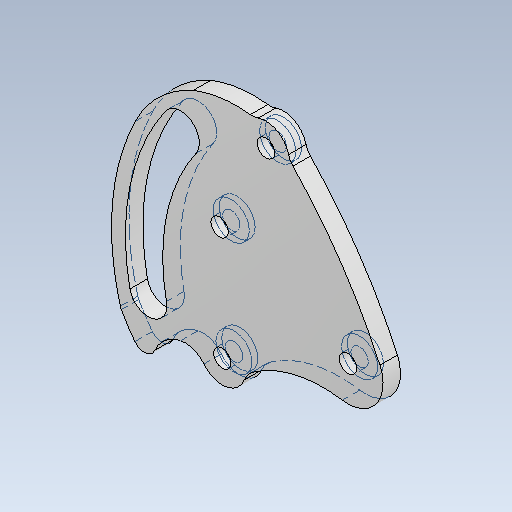
# Autodesk Inventor part: アンノーン前
Saved by Autodesk Inventor 2020 (Build 240168000, 168)
## iProperties
Created: 2021-02-23
Part Number: アンノーン前
Material: アルミニウム 2014-T4
Document SubType Name: Modeling
Designer: AA19065
Density: 2.8 g/cm^3
Appearance: サテン
Mass: 9.74033 g
Surface Area: 32.1311 cm^2
Volume: 3.47869 cm^3
Author: AA19065
Autodesk Inventor part; units mm, degrees
ref_plane "YZ Plane" through (0, 0, 0) normal (1, 0, 0) x (0, 1, 0)
ref_plane "XZ Plane" through (0, 0, 0) normal (0, 1, 0) x (-1, 0, 0)
ref_plane "XY Plane" through (0, 0, 0) normal (0, 0, 1) x (1, 0, 0)
sketch "スケッチ1" plane through (0, 0, 0) normal (0, 0, 1) x (1, 0, 0)
  line L0 (108, 72.831817) -> (108, -27.637331) construction
  circle A0 centre (90, 27) radius 3
  circle A1 centre (104.07345, 2) radius 6.025
  circle A2 centre (90, 27) radius 1.5
  circle A3 centre (104.07345, 2) radius 1.5
  circle A4 centre (82.04031, 11.281864) radius 1.5
  circle A5 centre (82.5, -8) radius 3
  circle A6 centre (82.5, -8) radius 1.5
  arc A7 (66.645247, -5.64) -> (72.915941, -4.36) centre (69.780594, -5) ccw
  arc A8 (72.724551, 23.828571) -> (66.645247, -5.64) centre (104.07345, 2) ccw
  arc A9 (77.976723, 20.171429) -> (72.915941, -4.36) centre (104.07345, 2) ccw
  arc A10 (77.976723, 20.171429) -> (72.724551, 23.828571) centre (75.350637, 22) ccw
  circle A11 centre (137.322151, 20) radius 1.25
  circle A12 centre (133.5, -8) radius 3
  circle A13 centre (133.5, -8) radius 1.5
  circle A14 centre (146, 10) radius 1.5
  arc A15 (-6.089587, 13.373015) -> (73.990447, 1.93301) centre (42.288654, 66.020578) ccw construction
  line L1 (108, 72.831817) -> (108, -27.637331) construction
  arc A16 (142.009553, 1.93301) -> (222.089587, 13.373015) centre (173.711346, 66.020578) ccw construction
  arc A17 (142.29705, -19.072921) -> (142.660887, 27.253552) centre (125.709293, 4.222021) ccw
  arc A18 (136.80781, 35.127338) -> (180.06622, 10.718677) centre (180.861669, 62.665248) ccw
  circle A19 centre (137.322151, 20) radius 9.006449
  arc A20 (128.322651, 20.353731) -> (130.555913, -8.5765) centre (253.226204, 15.444317) ccw
  arc A21 (133.414591, -10.998784) -> (152.948723, -4.485529) centre (134.268683, 18.989056) ccw
  arc A22 (35.93378, 10.718677) -> (79.19219, 35.127338) centre (35.138331, 62.665248) ccw
  arc A23 (73.339113, 27.253552) -> (73.70295, -19.072921) centre (90.290707, 4.222021) ccw
  arc A24 (90.887703, 29.865656) -> (71.118535, 25.188537) centre (84.969685, 10.761283) ccw
  arc A25 (109.559222, 4.491371) -> (92.075879, 29.165808) centre (36.719095, -28.589074) ccw
  arc A26 (80.567193, -10.294397) -> (70.653319, -16.566942) centre (76.603177, -15) ccw
  circle A27 centre (76.603177, -15) radius 5 construction
  circle A28 centre (94, -11) radius 1.5
  circle A29 centre (94, -11) radius 3
  arc A30 (103.111347, -3.947687) -> (84.657245, -10.084777) centre (99.757959, -24.678215) ccw
  point P0 (0, 0)
  point P1 (0, 0)
  point P2 (153.490711, -2.560367)
  point P3 (70.420594, -8.135347)
  point P4 (68.814065, 23.104865)
  dimension "d0" = 2
  dimension "d1" = 30
  dimension "d2" = 125
  dimension "d3" = 80
  dimension "d4" = 20
  dimension "d5" = 6
  dimension "d6" = 21
  constraints: 47 point on circle, 30 centre point, 10 tangent, 4 end point, 3 symmetric about line, 1 coincident, 1 vertical, 32 other
  measures "d0" distance of point (153.491, -2.56) A21.end
  measures "d1" radius of A21
  measures "d2" radius of A20
  measures "d3" radius of A25
  measures "d4" radius of A24
  measures "d5" diameter of A29
  measures "d6" radius of A30
extrude "押し出し1" add sketch "スケッチ1" along normal blind 3 contours A0 | A0 A25 A1 A30 A5 A26 A23 A22 A24 | A1 | A5
fillet "フィレット1" radius 5 1 edges at (68.8141, 23.1049, 1.5)
fillet "フィレット2" radius 2 1 edges at (70.6533, -16.5669, 1.5)
sketch "スケッチ2" plane through (0, 0, 0) normal (0, 0, -1) x (-1, 0, 0)
  circle A0 centre (-82.04031, 11.281864) radius 1.5
  arc A1 (-70.932275, -12.613165) -> (-67.494617, -13.044892) centre (-69.088898, -11.837303) ccw
  arc A2 (-67.494617, -13.044892) -> (-68.54743, 22.797215) centre (-90.290707, 4.222021) ccw
  arc A3 (-68.54743, 22.797215) -> (-69.082243, 23.334729) centre (-72.349055, 19.549502) ccw
  arc A4 (-71.118535, 25.188537) -> (-69.082243, 23.334729) centre (-35.138331, 62.665248) ccw
  arc A5 (-71.118535, 25.188537) -> (-90.887703, 29.865656) centre (-84.969685, 10.761283) ccw
  arc A6 (-90.887703, 29.865656) -> (-92.075879, 29.165808) centre (-90, 27) ccw
  arc A7 (-92.075879, 29.165808) -> (-109.559222, 4.491371) centre (-36.719095, -28.589074) ccw
  arc A8 (-109.559222, 4.491371) -> (-103.111347, -3.947687) centre (-104.07345, 2) ccw
  arc A9 (-84.657245, -10.084777) -> (-103.111347, -3.947687) centre (-99.757959, -24.678215) ccw
  arc A10 (-84.657245, -10.084777) -> (-80.567193, -10.294397) centre (-82.5, -8) ccw
  arc A11 (-70.932275, -12.613165) -> (-80.567193, -10.294397) centre (-76.603177, -15) ccw
  circle A12 centre (-82.5, -8) radius 1.5
  circle A13 centre (-104.07345, 2) radius 1.5
  circle A14 centre (-90, 27) radius 1.5
  circle A15 centre (-82.04031, 11.281864) radius 1.5
  arc A16 (-72.724551, 23.828571) -> (-77.976723, 20.171429) centre (-75.350637, 22) ccw
  arc A17 (-66.645247, -5.64) -> (-72.724551, 23.828571) centre (-104.07345, 2) ccw
  arc A18 (-72.915941, -4.36) -> (-66.645247, -5.64) centre (-69.780594, -5) ccw
  arc A19 (-72.915941, -4.36) -> (-77.976723, 20.171429) centre (-104.07345, 2) ccw
  circle A20 centre (-90, 27) radius 3.1
  circle A21 centre (-82.04031, 11.281864) radius 3.1
  circle A22 centre (-104.07345, 2) radius 3.1
  circle A23 centre (-82.5, -8) radius 3.1
  arc A24 (-86.256515, -9.37426) -> (-87.720107, -7.470946) centre (-90.013031, -10.748521) ccw
  arc A25 (-86.256515, -9.37426) -> (-79.334786, -10.445694) centre (-82.5, -8) ccw
  arc A26 (-75.363887, -8.973369) -> (-79.334786, -10.445694) centre (-76.169572, -12.891388) ccw
  arc A27 (-70.932275, -12.613165) -> (-80.567193, -10.294397) centre (-76.603177, -15) ccw
  arc A28 (-94.623726, 26.61105) -> (-93.882942, 27.960603) centre (-96.795149, 28.681055) ccw
  arc A29 (-88.670242, 30.772498) -> (-93.882942, 27.960603) centre (-90, 27) ccw
  arc A30 (-88.670242, 30.772498) -> (-87.320327, 30.622665) centre (-87.672923, 33.601872) ccw
  point P0 (0, 0)
  dimension "d11" = 6.2
  dimension "d12" = 6.2
  dimension "d13" = 6.2
  dimension "d14" = 6.2
  dimension "d15" = 4
  dimension "d16" = 4
  dimension "d17" = 4
  dimension "d18" = 4
  dimension "d19" = 3
  dimension "d20" = 3
  constraints: 16 point on circle, 10 centre point, 8 tangent, 4 coincident, 2 concentric
  measures "d11" diameter of A20
  measures "d12" diameter of A21
  measures "d13" diameter of A22
  measures "d14" diameter of A23
  measures "d15" radius of A25
  measures "d16" radius of A26
  measures "d17" radius of A24
  measures "d18" radius of A29
  measures "d19" radius of A30
  measures "d20" radius of A28
extrude "押し出し2" add sketch "スケッチ2" against normal up to surface (3 mm away) contours A26 A25 A24 A9 A23 A11 | A23 A9 A10 A11 | A5 A20 A7 A28 A29 A30 | A5 A6 A7 A20 picked at (-81.994217, -10.979131) picked at (-91.467973, 29.678904)
extrude "押し出し3" cut sketch "スケッチ2" against normal blind 1 contours A23 A9 A10 A11 | A11 A10 A9 A23 | A20 A7 A6 A5 | A5 A6 A7 A20 | A12 | A14 | A21 | A22
sketch "スケッチ4" plane through (0, 0, 3) normal (0, 0, 1) x (1, 0, 0)
  arc A0 (67.494617, -13.044892) -> (70.932275, -12.613165) centre (69.088898, -11.837303) ccw
  arc A1 (75.363887, -8.973369) -> (70.932275, -12.613165) centre (76.603177, -15) ccw
  arc A2 (79.334786, -10.445694) -> (75.363887, -8.973369) centre (76.169572, -12.891388) ccw
  arc A3 (79.334786, -10.445694) -> (86.256515, -9.37426) centre (82.5, -8) ccw
  arc A4 (87.720107, -7.470946) -> (86.256515, -9.37426) centre (90.013031, -10.748521) ccw
  arc A5 (103.111347, -3.947687) -> (87.720107, -7.470946) centre (99.757959, -24.678215) ccw
  arc A6 (103.111347, -3.947687) -> (109.559222, 4.491371) centre (104.07345, 2) ccw
  arc A7 (109.559222, 4.491371) -> (94.623726, 26.61105) centre (36.719095, -28.589074) ccw
  arc A8 (93.882942, 27.960603) -> (94.623726, 26.61105) centre (96.795149, 28.681055) ccw
  arc A9 (93.882942, 27.960603) -> (88.670242, 30.772498) centre (90, 27) ccw
  arc A10 (87.320327, 30.622665) -> (88.670242, 30.772498) centre (87.672923, 33.601872) ccw
  arc A11 (87.320327, 30.622665) -> (71.118535, 25.188537) centre (84.969685, 10.761283) ccw
  arc A12 (69.082243, 23.334729) -> (71.118535, 25.188537) centre (35.138331, 62.665248) ccw
  arc A13 (69.082243, 23.334729) -> (68.54743, 22.797215) centre (72.349055, 19.549502) ccw
  arc A14 (68.54743, 22.797215) -> (67.494617, -13.044892) centre (90.290707, 4.222021) ccw
  circle A15 centre (82.5, -8) radius 1.5
  circle A16 centre (104.07345, 2) radius 1.5
  circle A17 centre (90, 27) radius 1.5
  circle A18 centre (82.04031, 11.281864) radius 1.5
  arc A19 (77.976723, 20.171429) -> (72.724551, 23.828571) centre (75.350637, 22) ccw
  arc A20 (77.976723, 20.171429) -> (72.915941, -4.36) centre (104.07345, 2) ccw
  arc A21 (66.645247, -5.64) -> (72.915941, -4.36) centre (69.780594, -5) ccw
  arc A22 (72.724551, 23.828571) -> (66.645247, -5.64) centre (104.07345, 2) ccw
  arc A23 (70.112674, 24.248139) -> (65.061877, -9.243272) centre (104.07345, 2) ccw
  arc A24 (72.724551, 23.828571) -> (66.645247, -5.64) centre (104.07345, 2) ccw
  arc A25 (77.522944, 29.323235) -> (67.556607, 19.743566) centre (85.545451, 11.002771) ccw
  point P0 (0, 0)
  dimension "d28" = 20
  constraints: 8 point on circle, 2 centre point, 1 concentric, 1 tangent
  measures "d28" radius of A25
sketch "スケッチ4 outline for 押し出し4" plane through (0, 0, 3) normal (0, 0, 1) x (1, 0, 0)
  arc A0 (69.082243, 23.334729) -> (68.54743, 22.797215) centre (72.349055, 19.549502) ccw
  arc A1 (68.54743, 22.797215) -> (65.061877, -9.243272) centre (90.290707, 4.222021) ccw
  arc A2 (65.061877, -9.243272) -> (67.556607, 19.743566) centre (104.07345, 2) cw
  arc A3 (67.556607, 19.743566) -> (77.522944, 29.323235) centre (85.545451, 11.002771) cw
  arc A4 (77.522944, 29.323235) -> (71.118535, 25.188537) centre (84.969685, 10.761283) ccw
  arc A5 (71.118535, 25.188537) -> (69.082243, 23.334729) centre (35.138331, 62.665248) cw
extrude "押し出し4" cut sketch "スケッチ4 outline for 押し出し4" against normal blind 10
fillet "フィレット3" radius 2 1 edges at (65.0619, -9.2433, 1.5)
